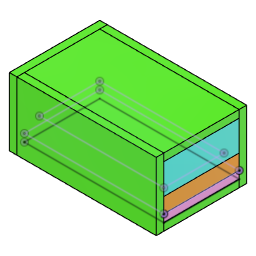
Mini apple boxes v15 (Autodesk Fusion 360 design; units mm, degrees)
Autodesk Fusion 360 part; units mm, degrees
sketch "p_sketch" plane through (0, 0, 0) normal (0, 1, 0) x (1, 0, 0) in component "pancake"
  line L0 (0, 0) -> (117.475, 0)
  line L1 (117.475, 0) -> (117.475, 63.5)
  line L2 (117.475, 63.5) -> (0, 63.5)
  line L3 (0, 63.5) -> (0, 0)
  dimension "d1" = 117.475
  dimension "d2" = 63.5
  constraint horizontal L0
  constraint vertical L1
  constraint horizontal L2
  constraint vertical L3
  constraint coincident L0.start L3.end
  measures "d1" distance of L1.end L2.end
  measures "d2" distance of L0.end L1.end
extrude "Extrude1" add sketch "p_sketch" along normal blind 6.35 makes body 1 in component "pancake"
sketch "q_mainBodySketch" plane through (0, 6.35, 0) normal (0, 1, 0) x (-1, 0, 0) in component "quarter"
  line L0 (0, -63.5) -> (0, 0)
  line L1 (0, 0) -> (-117.475, 0)
  line L2 (-117.475, 0) -> (-117.475, -63.5)
  line L3 (-117.475, -63.5) -> (0, -63.5)
extrude "Extrude1'" add sketch "q_mainBodySketch" along normal blind 12.7 separate body makes body 2 in component "quarter"
move_face "OffsetFaces1" offset -6.35 1 faces at (117.475, 10.5833, -42.3333) on bodies 2 in component "quarter"
move_face "OffsetFaces2" offset -6.35 1 faces at (0, 14.8167, -21.1667) on bodies 2 in component "quarter"
sketch "q_endSketch" plane through (111.125, 0, 0) normal (1, 0, 0) x (0, 0, -1) in component "quarter"
  line L0 (0, 6.35) -> (63.5, 6.35)
  line L1 (63.5, 6.35) -> (63.5, 19.05)
  line L2 (63.5, 19.05) -> (0, 19.05)
  line L3 (0, 19.05) -> (0, 6.35)
extrude "Extrude2" add sketch "q_endSketch" along normal blind 6.35 separate body makes body 3 in component "quarter"
ref_plane "WorkPlane1" through (58.7375, 12.7, -31.75) normal (1, 0, 0) x (0, 0, -1) in component "quarter"
mirror "Mirror1" about plane through (58.7375, 12.7, -31.75) normal (1, 0, 0) of bodies 3 makes body 4 in component "quarter"
move_face "OffsetFaces3" offset -6.35 2 faces at (76.2, 14.8167, 0) (41.275, 14.8167, -63.5) on bodies 2 in component "quarter"
ref_plane "WorkPlane2" through (58.7375, 12.7, -31.75) normal (0, 0, 1) x (1, 0, 0) in component "quarter"
sketch "q_sideSketch" plane through (0, 0, -6.35) normal (0, 0, 1) x (1, 0, 0) in component "quarter"
  line L0 (6.35, 6.35) -> (111.125, 6.35)
  line L1 (111.125, 6.35) -> (111.125, 19.05)
  line L2 (111.125, 19.05) -> (6.35, 19.05)
  line L3 (6.35, 19.05) -> (6.35, 6.35)
  line L4 (6.35, 19.05) -> (111.125, 19.05)
  line L5 (111.125, 19.05) -> (111.125, 6.35)
  line L6 (111.125, 6.35) -> (6.35, 6.35)
  line L7 (6.35, 6.35) -> (6.35, 19.05)
  constraint horizontal L4
  constraint vertical L5
  constraint horizontal L6
  constraint vertical L7
  constraint coincident L0.end L1.start
  constraint coincident L2.end L3.start
extrude "Extrude3" add sketch "q_sideSketch" along normal blind 6.35 separate body makes body 5 in component "quarter"
mirror "Mirror2" about plane through (58.7375, 12.7, -31.75) normal (0, 0, 1) of bodies 5 makes body 6 in component "quarter"
sketch "h_mainBody" plane through (0, 19.05, 0) normal (0, 1, 0) x (-1, 0, 0) in component "half"
  line L0 (-111.125, -57.15) -> (-6.35, -57.15)
  line L1 (-6.35, -57.15) -> (-6.35, -6.35)
  line L2 (-6.35, -6.35) -> (-111.125, -6.35)
  line L3 (-111.125, -6.35) -> (-111.125, -57.15)
  line L4 (0, -63.5) -> (0, 0)
  line L5 (-6.35, -63.5) -> (0, -63.5)
  line L6 (-111.125, -63.5) -> (-6.35, -63.5)
  line L7 (-111.125, -63.5) -> (-117.475, -63.5)
  line L8 (-117.475, -63.5) -> (-117.475, 0)
  line L9 (-111.125, 0) -> (-117.475, 0)
  line L10 (-111.125, 0) -> (-6.35, 0)
  line L11 (-6.35, 0) -> (0, 0)
  line L12 (0, 0) -> (-117.475, 0)
  line L13 (-117.475, 0) -> (-117.475, -63.5)
  line L14 (-117.475, -63.5) -> (0, -63.5)
  line L15 (0, -63.5) -> (0, 0)
  constraint horizontal L12
  constraint vertical L13
  constraint horizontal L14
  constraint vertical L15
  constraint coincident L7.end L8.start
  constraint coincident L4.end L11.end
extrude "Extrude1''" add sketch "h_mainBody" along normal blind 25.4 separate body contours L0 L1 L2 L3 | L4 L5 L6 L7 L8 L9 L10 L11 L12 L13 L14 L15 makes body 7 in component "half"
move_face "OffsetFaces1'" offset -6.35 2 faces at (117.475, 27.5167, -42.3333) (0, 27.5167, -42.3333) on bodies 7 in component "half"
move_face "OffsetFaces2'" offset -6.35 2 faces at (41.275, 35.9833, 0) (41.275, 35.9833, -63.5) on bodies 7 in component "half"
sketch "h_centerCut" plane through (111.125, 0, 0) normal (1, 0, 0) x (0, 0, -1) in component "half"
  line L0 (6.35, 19.05) -> (57.15, 19.05)
  line L1 (57.15, 19.05) -> (57.15, 44.45)
  line L2 (57.15, 44.45) -> (6.35, 44.45)
  line L3 (6.35, 44.45) -> (6.35, 19.05)
  line L4 (6.35, 38.1) -> (57.15, 38.1)
  line L5 (57.15, 38.1) -> (57.15, 25.4)
  line L6 (57.15, 25.4) -> (6.35, 25.4)
  line L7 (6.35, 25.4) -> (6.35, 38.1)
  dimension "d22" = 6.35
  dimension "d23" = 6.35
  constraint horizontal L4
  constraint vertical L5
  constraint horizontal L6
  constraint vertical L7
  constraint coincident L3 L4.start
  constraint coincident L1 L4.end
  measures "d22" vertical distance of L1.end L4.end
  measures "d23" vertical distance of L0.end L5.end
extrude "Extrude2'" cut sketch "h_centerCut" against normal blind 104.775 contours L1 L3 L4 L5 L6 L7 bodies 7 makes body 8 at (41.275, 19.05, -40.2167) in component "half"
sketch "h_endSketch" plane through (111.125, 0, 0) normal (1, 0, 0) x (0, 0, -1) in component "half"
  line L0 (6.35, 38.1) -> (57.15, 38.1)
  line L1 (57.15, 38.1) -> (57.15, 44.45)
  line L2 (57.15, 44.45) -> (6.35, 44.45)
  line L3 (6.35, 44.45) -> (6.35, 38.1)
  line L4 (57.15, 25.4) -> (6.35, 25.4)
  line L5 (6.35, 25.4) -> (6.35, 19.05)
  line L6 (6.35, 19.05) -> (57.15, 19.05)
  line L7 (57.15, 19.05) -> (57.15, 25.4)
  line L8 (0, 19.05) -> (0, 6.35)
  line L9 (0, 6.35) -> (63.5, 6.35)
  line L10 (63.5, 6.35) -> (63.5, 19.05)
  line L11 (63.5, 19.05) -> (0, 19.05)
  line L12 (63.5, 44.45) -> (0, 44.45)
  line L13 (0, 44.45) -> (0, 19.05)
  line L14 (0, 19.05) -> (63.5, 19.05)
  line L15 (63.5, 19.05) -> (63.5, 44.45)
  constraint horizontal L12
  constraint vertical L13
  constraint horizontal L14
  constraint vertical L15
  constraint coincident L8.start L11.end
  constraint coincident L10.end L11.start
  constraint coincident L2 L12.start
extrude "Extrude3'" add sketch "h_endSketch" along normal blind 6.35 separate body contours L0 L1 L2 L3 L12 | L0 L1 L3 L4 L5 L7 L11 L12 L13 L14 L15 | L4 L5 L6 L7 L11 L14 makes body 9 in component "half"
ref_plane "WorkPlane1" through (58.7375, 41.275, -31.75) normal (1, 0, 0) x (0, 0, -1) in component "half"
mirror "Mirror1'" about plane through (58.7375, 41.275, -31.75) normal (1, 0, 0) of bodies 9 makes body 10 in component "half"
ref_plane "WorkPlane2" through (58.7375, 41.275, -31.75) normal (0, 0, 1) x (1, 0, 0) in component "half"
sketch "h_sides" plane through (0, 0, -6.35) normal (0, 0, 1) x (1, 0, 0) in component "half"
  line L0 (6.35, 38.1) -> (111.125, 38.1)
  line L1 (111.125, 38.1) -> (111.125, 44.45)
  line L2 (111.125, 44.45) -> (6.35, 44.45)
  line L3 (6.35, 44.45) -> (6.35, 38.1)
  line L4 (111.125, 25.4) -> (6.35, 25.4)
  line L5 (6.35, 25.4) -> (6.35, 19.05)
  line L6 (6.35, 19.05) -> (111.125, 19.05)
  line L7 (111.125, 19.05) -> (111.125, 25.4)
  line L8 (6.35, 44.45) -> (111.125, 44.45)
  line L9 (111.125, 44.45) -> (111.125, 19.05)
  line L10 (111.125, 19.05) -> (6.35, 19.05)
  line L11 (6.35, 19.05) -> (6.35, 44.45)
  constraint horizontal L8
  constraint vertical L9
  constraint horizontal L10
  constraint vertical L11
  constraint coincident L6.end L7.start
  constraint coincident L2.end L3.start
extrude "Extrude4" add sketch "h_sides" along normal blind 6.35 separate body makes body 11 in component "half"
mirror "Mirror2'" about plane through (58.7375, 41.275, -31.75) normal (0, 0, 1) of bodies 11 makes body 12 in component "half"
sketch "Sketch5" plane through (0, 0, -6.35) normal (0, 0, -1) x (-1, 0, 0) in component "half"
  line L0 (-111.125, 19.05) -> (-6.35, 19.05)
  line L1 (-6.35, 19.05) -> (-6.35, 44.45)
  line L2 (-6.35, 44.45) -> (-111.125, 44.45)
  line L3 (-111.125, 44.45) -> (-111.125, 19.05)
  line L4 (-111.125, 38.1) -> (-6.35, 38.1)
  line L5 (-6.35, 38.1) -> (-6.35, 44.45)
  line L6 (-6.35, 44.45) -> (-111.125, 44.45)
  line L7 (-111.125, 44.45) -> (-111.125, 38.1)
  line L8 (-6.35, 25.4) -> (-111.125, 25.4)
  line L9 (-111.125, 25.4) -> (-111.125, 19.05)
  line L10 (-111.125, 19.05) -> (-6.35, 19.05)
  line L11 (-6.35, 19.05) -> (-6.35, 25.4)
  line L12 (-65.0875, 38.1) -> (-58.7375, 38.1)
  line L13 (-58.7375, 38.1) -> (-58.7375, 25.4)
  line L14 (-58.7375, 25.4) -> (-65.0875, 25.4)
  line L15 (-65.0875, 25.4) -> (-65.0875, 38.1)
  dimension "d34" = 6.35
  dimension "d35" = 46.0375
  constraint horizontal L12
  constraint vertical L13
  constraint horizontal L14
  constraint vertical L15
  constraint coincident L8 L13.end
  constraint coincident L4 L12.end
  measures "d34" distance of L12.start L12.end
  measures "d35" distance of L4.start L12.start
extrude "Extrude5" add sketch "Sketch5" along normal blind 50.8 separate body contours L4 L8 L12 L13 L14 L15 makes body 13 in component "half"
sketch "f_endSketch" plane through (117.475, 0, 0) normal (1, 0, 0) x (0, 0, -1) in component "full"
  line L0 (63.5, 19.05) -> (63.5, 44.45)
  line L1 (63.5, 44.45) -> (0, 44.45)
  line L2 (0, 44.45) -> (0, 19.05)
  line L3 (0, 19.05) -> (63.5, 19.05)
  line L4 (0, 0) -> (63.5, 0)
  line L5 (63.5, 0) -> (63.5, 6.35)
  line L6 (63.5, 6.35) -> (0, 6.35)
  line L7 (0, 6.35) -> (0, 0)
  line L8 (0, 19.05) -> (0, 6.35)
  line L9 (0, 6.35) -> (63.5, 6.35)
  line L10 (63.5, 6.35) -> (63.5, 19.05)
  line L11 (63.5, 19.05) -> (0, 19.05)
  line L12 (-6.35, 50.8) -> (69.85, 50.8)
  line L13 (69.85, 50.8) -> (69.85, -6.35)
  line L14 (69.85, -6.35) -> (-6.35, -6.35)
  line L15 (-6.35, -6.35) -> (-6.35, 50.8)
  dimension "d38" = 6.35
  dimension "d39" = 6.35
  dimension "d40" = 6.35
  dimension "d41" = 6.35
  constraint horizontal L12
  constraint vertical L13
  constraint horizontal L14
  constraint vertical L15
  measures "d38" vertical distance of L0.end L12.end
  measures "d39" vertical distance of L4.end L13.end
  measures "d40" horizontal distance of L0.end L12.end
  measures "d41" horizontal distance of L1.end L12.start
extrude "Extrude1'''" add sketch "f_endSketch" along normal blind 6.35 separate body contours L0 L1 L2 L3 L11 | L3 L6 L8 L9 L10 L11 | L4 L5 L6 L7 L9 | L12 L13 L14 L15 makes body 14 in component "full"
ref_plane "WorkPlane1" through (58.7375, 31.75, -31.75) normal (1, 0, 0) x (0, 0, -1) in component "full"
mirror "Mirror1''" about plane through (58.7375, 31.75, -31.75) normal (1, 0, 0) of bodies 14 makes body 15 in component "full"
sketch "f_sideSketch" plane through (0, 0, 0) normal (0, 0, 1) x (1, 0, 0) in component "full"
  line L0 (6.35, 19.05) -> (111.125, 19.05)
  line L1 (111.125, 19.05) -> (111.125, 44.45)
  line L2 (111.125, 44.45) -> (6.35, 44.45)
  line L3 (6.35, 44.45) -> (6.35, 19.05)
  line L4 (6.35, 19.05) -> (6.35, 44.45)
  line L5 (6.35, 44.45) -> (0, 44.45)
  line L6 (0, 44.45) -> (0, 19.05)
  line L7 (0, 19.05) -> (6.35, 19.05)
  line L8 (6.35, 6.35) -> (6.35, 19.05)
  line L9 (6.35, 19.05) -> (0, 19.05)
  line L10 (0, 19.05) -> (0, 6.35)
  line L11 (0, 6.35) -> (6.35, 6.35)
  line L12 (0, 0) -> (117.475, 0)
  line L13 (117.475, 0) -> (117.475, 6.35)
  line L14 (117.475, 6.35) -> (0, 6.35)
  line L15 (0, 6.35) -> (0, 0)
  line L16 (6.35, 6.35) -> (111.125, 6.35)
  line L17 (111.125, 6.35) -> (111.125, 19.05)
  line L18 (111.125, 19.05) -> (6.35, 19.05)
  line L19 (6.35, 19.05) -> (6.35, 6.35)
  line L20 (111.125, 44.45) -> (111.125, 19.05)
  line L21 (111.125, 19.05) -> (117.475, 19.05)
  line L22 (117.475, 19.05) -> (117.475, 44.45)
  line L23 (117.475, 44.45) -> (111.125, 44.45)
  line L24 (111.125, 19.05) -> (111.125, 6.35)
  line L25 (111.125, 6.35) -> (117.475, 6.35)
  line L26 (117.475, 6.35) -> (117.475, 19.05)
  line L27 (117.475, 19.05) -> (111.125, 19.05)
  line L28 (123.825, 50.8) -> (123.825, -6.35)
  line L29 (0, -6.35) -> (0, 50.8)
  line L30 (0, 50.8) -> (-6.35, 50.8)
  line L31 (-6.35, 50.8) -> (-6.35, -6.35)
  line L32 (-6.35, -6.35) -> (0, -6.35)
  line L33 (0, 50.8) -> (117.475, 50.8)
  line L34 (117.475, 50.8) -> (117.475, -6.35)
  line L35 (117.475, -6.35) -> (0, -6.35)
  line L36 (0, -6.35) -> (0, 50.8)
  point P0 (117.475, -6.35)
  constraint horizontal L33
  constraint vertical L34
  constraint horizontal L35
  constraint vertical L36
  constraint coincident L29.end L30.start
  constraint coincident P0 L34.end
extrude "Extrude2''" add sketch "f_sideSketch" along normal blind 6.35 separate body contours L0 L1 L2 L3 L4 L18 L20 | L3 L4 L5 L6 L7 L9 L29 L36 | L7 L8 L9 L10 L11 L14 L19 L29 L36 | L0 L8 L14 L16 L17 L18 L19 L24 | L14 L17 L21 L24 L25 L26 L27 L34 | L1 L20 L21 L22 L23 L27 L34 | L2 L5 L23 L29 L33 L34 L36 | L11 L12 L13 L14 L15 L16 L25 L29 L34 L36 | L12 L29 L34 L35 L36 makes body 16 in component "full"
ref_plane "WorkPlane2" through (58.7375, 31.75, -31.75) normal (0, 0, 1) x (1, 0, 0) in component "full"
mirror "Mirror2''" about plane through (58.7375, 31.75, -31.75) normal (0, 0, 1) of bodies 16 makes body 17 in component "full"
ref_plane "WorkPlane3" through (58.7375, 22.225, -31.75) normal (0, 1, 0) x (0, 0, 1) in component "full"
sketch "f_topSketch" plane through (0, 0, 0) normal (0, -1, 0) x (1, 0, 0) in component "full"
  line L0 (0, 0) -> (0, -63.5)
  line L1 (0, -63.5) -> (117.475, -63.5)
  line L2 (117.475, -63.5) -> (117.475, 0)
  line L3 (117.475, 0) -> (0, 0)
  line L4 (0, 0) -> (117.475, 0)
  line L5 (117.475, 0) -> (117.475, -63.5)
  line L6 (117.475, -63.5) -> (0, -63.5)
  line L7 (0, -63.5) -> (0, 0)
  constraint horizontal L4
  constraint vertical L5
  constraint horizontal L6
  constraint vertical L7
  constraint coincident L1.end L2.start
  constraint coincident L0.start L3.end
extrude "Extrude3''" add sketch "f_topSketch" along normal blind 6.35 separate body makes body 18 in component "full"
mirror "Mirror3" about plane through (58.7375, 22.225, -31.75) normal (0, 1, 0) of bodies 18 makes body 19 in component "full"
sketch "Sketch4" plane through (-6.35, 0, 0) normal (-1, 0, 0) x (0, 0, 1) in component "full"
  line L0 (-69.85, -6.35) -> (6.35, -6.35)
  line L1 (6.35, -6.35) -> (6.35, 50.8)
  line L2 (6.35, 50.8) -> (-69.85, 50.8)
  line L3 (-69.85, 50.8) -> (-69.85, -6.35)
  line L4 (-50.8, 28.575) -> (-12.7, 28.575)
  line L5 (-12.7, 28.575) -> (-12.7, 15.875)
  line L6 (-12.7, 15.875) -> (-50.8, 15.875)
  line L7 (-50.8, 15.875) -> (-50.8, 28.575)
  arc A0 (-12.7, 15.875) -> (-12.7, 28.575) centre (-12.7, 22.225) ccw
  arc A1 (-50.8, 28.575) -> (-50.8, 15.875) centre (-50.8, 22.225) ccw
  dimension "d54" = 12.7
  dimension "d55" = 19.05
  dimension "d56" = 19.05
  dimension "d57" = 22.225
  constraint horizontal L4
  constraint vertical L5
  constraint horizontal L6
  constraint vertical L7
  constraint midpoint L5 A0.centre
  constraint midpoint L7 A1.centre
  measures "d54" distance of L4.end L5.end
  measures "d55" horizontal distance of L1.end L4.end
  measures "d56" horizontal distance of L2.end L4.start
  measures "d57" vertical distance of L1.end L4.end
extrude "Extrude4'" cut sketch "Sketch4" against normal blind 6.35 contours L4 L5 L6 L7 | L7 A1 | L5 A0 bodies 15 in component "full"
sketch "q_topBottom" plane through (0, 19.05, 0) normal (0, 1, 0) x (-1, 0, 0) in component "quarter"
  line L0 (-111.125, -57.15) -> (-6.35, -57.15)
  line L1 (-6.35, -57.15) -> (-6.35, -6.35)
  line L2 (-6.35, -6.35) -> (-111.125, -6.35)
  line L3 (-111.125, -6.35) -> (-111.125, -57.15)
sketch "h_topBottom" plane through (0, 44.45, 0) normal (0, 1, 0) x (-1, 0, 0) in component "half"
  line L0 (-6.35, -57.15) -> (-6.35, -6.35)
  line L1 (-6.35, -6.35) -> (-111.125, -6.35)
  line L2 (-111.125, -6.35) -> (-111.125, -57.15)
  line L3 (-111.125, -57.15) -> (-6.35, -57.15)
sketch "f_capExport" plane through (-6.35, 0, 0) normal (-1, 0, 0) x (0, 0, 1) in component "laserExports"
  line L0 (-50.8, 28.575) -> (-12.7, 28.575)
  arc A0 (-12.7, 15.875) -> (-12.7, 28.575) centre (-12.7, 22.225) ccw
  line L1 (-12.7, 15.875) -> (-50.8, 15.875)
  arc A1 (-50.8, 28.575) -> (-50.8, 15.875) centre (-50.8, 22.225) ccw
  line L2 (-69.85, -6.35) -> (6.35, -6.35)
  line L3 (6.35, -6.35) -> (6.35, 50.8)
  line L4 (6.35, 50.8) -> (-69.85, 50.8)
  line L5 (-69.85, 50.8) -> (-69.85, -6.35)
sketch "f_sidesExport" plane through (0, 0, 6.35) normal (0, 0, 1) x (1, 0, 0) in component "laserExports"
  line L0 (0, -6.35) -> (117.475, -6.35)
  line L1 (117.475, -6.35) -> (117.475, 50.8)
  line L2 (117.475, 50.8) -> (0, 50.8)
  line L3 (0, 50.8) -> (0, -6.35)
sketch "f_topBottomEport" plane through (0, 50.8, 0) normal (0, 1, 0) x (-1, 0, 0) in component "laserExports"
  line L0 (-117.475, -63.5) -> (0, -63.5)
  line L1 (0, -63.5) -> (0, 0)
  line L2 (0, 0) -> (-117.475, 0)
  line L3 (-117.475, 0) -> (-117.475, -63.5)
sketch "h_capExport" plane through (0, 0, 0) normal (-1, 0, 0) x (0, 0, 1) in component "laserExports"
  line L0 (-63.5, 44.45) -> (-63.5, 19.05)
  line L1 (-63.5, 19.05) -> (0, 19.05)
  line L2 (0, 19.05) -> (0, 44.45)
  line L3 (0, 44.45) -> (-63.5, 44.45)
sketch "h_SidesExport" plane through (0, 0, 0) normal (0, 0, 1) x (1, 0, 0) in component "laserExports"
  line L0 (6.35, 19.05) -> (111.125, 19.05)
  line L1 (111.125, 19.05) -> (111.125, 44.45)
  line L2 (111.125, 44.45) -> (6.35, 44.45)
  line L3 (6.35, 44.45) -> (6.35, 19.05)
sketch "h_topBottomExport" plane through (0, 44.45, 0) normal (0, 1, 0) x (-1, 0, 0) in component "laserExports"
  line L0 (-6.35, -57.15) -> (-6.35, -6.35)
  line L1 (-6.35, -6.35) -> (-111.125, -6.35)
  line L2 (-111.125, -6.35) -> (-111.125, -57.15)
  line L3 (-111.125, -57.15) -> (-6.35, -57.15)
sketch "q_capExport" plane through (0, 0, 0) normal (-1, 0, 0) x (0, 0, 1) in component "laserExports"
  line L0 (0, 6.35) -> (0, 19.05)
  line L1 (0, 19.05) -> (-63.5, 19.05)
  line L2 (-63.5, 19.05) -> (-63.5, 6.35)
  line L3 (-63.5, 6.35) -> (0, 6.35)
sketch "q_sidesExport" plane through (0, 0, 0) normal (0, 0, 1) x (1, 0, 0) in component "laserExports"
  line L0 (6.35, 6.35) -> (111.125, 6.35)
  line L1 (111.125, 6.35) -> (111.125, 19.05)
  line L2 (111.125, 19.05) -> (6.35, 19.05)
  line L3 (6.35, 19.05) -> (6.35, 6.35)
sketch "q_topBottomExport" plane through (58.7375, 19.05, -31.75) normal (0, 1, 0) x (-1, 0, 0) in component "laserExports"
  line L0 (-52.3875, -25.4) -> (52.3875, -25.4)
  line L1 (52.3875, -25.4) -> (52.3875, 25.4)
  line L2 (52.3875, 25.4) -> (-52.3875, 25.4)
  line L3 (-52.3875, 25.4) -> (-52.3875, -25.4)
sketch "p_Export" plane through (0, 6.35, 0) normal (0, 1, 0) x (-1, 0, 0) in component "laserExports"
  line L0 (0, -63.5) -> (0, 0)
  line L1 (0, 0) -> (-117.475, 0)
  line L2 (-117.475, 0) -> (-117.475, -63.5)
  line L3 (-117.475, -63.5) -> (0, -63.5)
component "pancake" placed x (1, 0, 0) y (0, 1, 0) z (0, 0, 1) at (0, 0, 0)
component "quarter" placed x (1, 0, 0) y (0, 1, 0) z (0, 0, 1) at (0, 0, 0)
component "half" placed x (1, 0, 0) y (0, 1, 0) z (0, 0, 1) at (0, 0, 0)
component "full" placed x (1, 0, 0) y (0, 1, 0) z (0, 0, 1) at (0, 0, 0)
component "laserExports" placed x (1, 0, 0) y (0, 1, 0) z (0, 0, 1) at (0, 0, 0)
hidden bodies 14
equation "d1 = ( 18.5 / 4 ) * 1 in"
equation "d2 = ( 10 / 4 ) * 1 in"
equation "d18 = 1\""
equation "d35 = ( ( 4.125 / 2 ) * 1 in ) - 0.25 in"
equation "d57 = ( 1.75 / 2 ) * 1 in"
named bodies: "p_mainBody", "q_mainBody", "q_end", "q_end (1)", "q_side1", "q_side2", "h_top", "h_bottom", "h_endcap1", "h_endcap2", "h_side1", "h_side2", "h_beam", "f_endcapUnused", "f_endcap", "f_side1", "f_side2", "f_bottom", "f_top"
